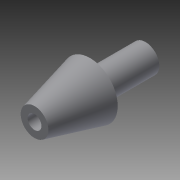
# Autodesk Inventor part: conver
Saved by Autodesk Inventor 2015 (Build 190159000, 159)
## iProperties
Created: 2014-11-30
Part Number: conver
Material: 常规
Document SubType Name: Modeling
Designer: zenkr
Density: 1 g/cm^3
Appearance: 默认
Author: zenkr
Autodesk Inventor part; units mm, degrees
ref_plane "YZ Plane" through (0, 0, 0) normal (1, 0, 0) x (0, 1, 0)
ref_plane "XY Plane" through (0, 0, 0) normal (0, 0, 1) x (1, 0, 0)
sketch "草图1" plane through (0, 0, 0) normal (0, 1, 0) x (-1, 0, 0)
  circle A0 centre (0, 0) radius 2
  dimension "d0" = 4
  constraints: 1 centre point, 1 coincident
  measures "d0" diameter of A0
ref_plane "工作平面1" through (0, -4, 0) normal (0, 1, 0) x (-1, 0, 0)
sketch "草图2" plane through (0, -4, 0) normal (0, 1, 0) x (-1, 0, 0)
  circle A0 centre (0, 0) radius 1
  dimension "d2" = 2
  constraints: 1 centre point, 1 coincident
  measures "d2" diameter of A0
loft "放样1" add profiles "草图1", "草图2"
sketch "草图3" plane through (0, 0, 0) normal (0, 1, 0) x (1, 0, 0)
  circle A0 centre (0, 0) radius 1
  dimension "d7" = 2
  constraints: 1 centre point, 1 coincident
  measures "d7" diameter of A0
extrude "拉伸1" add sketch "草图3" along normal blind 4
sketch "草图4" plane through (0, -4, 0) normal (0, 1, 0) x (-1, 0, 0)
  circle A0 centre (0, 0) radius 0.5
  dimension "d10" = 1
  constraints: 1 centre point, 1 coincident
  measures "d10" diameter of A0
extrude "拉伸2" cut sketch "草图4" along normal through all
